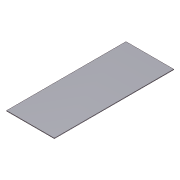
# Autodesk Inventor part: SpaceQuest_interconnect_3
Saved by Autodesk Inventor 2014 SP1 (Build 180222100, 222)
## iProperties
Created: 2013-06-08
Part Number: SpaceQuest_interconnect_3
Material: Stainless Steel
Document SubType Name: Modeling
Designer: Robert Davis
Mass: 0.01616 g
Surface Area: 0.814 cm^2
Volume: 0.002 cm^3
Density: 8.08 g/cm^3
Appearance: Steel
Author: Robert Davis
Autodesk Inventor part; units mm, degrees
ref_plane "YZ Plane" through (0, 0, 0) normal (1, 0, 0) x (0, 1, 0)
ref_plane "XZ Plane" through (0, 0, 0) normal (0, 1, 0) x (-1, 0, 0)
ref_plane "XY Plane" through (0, 0, 0) normal (0, 0, 1) x (1, 0, 0)
sketch "Sketch1" plane through (0, 0, 0) normal (0, 0, 1) x (1, 0, 0)
  line L0 (-2, 5) -> (2, 5)
  line L1 (2, 5) -> (2, -5)
  line L2 (2, -5) -> (-2, -5)
  line L3 (-2, -5) -> (-2, 5)
  line L4 (0, 0) -> (0, 1.6478)
  line L5 (0, 0) -> (2.3787, 0)
  dimension "d0" = 4
  dimension "d1" = 10
  constraints: 12 end point, 3 horizontal, 2 vertical, 1 coincident, 2 other
  measures "d0" distance of L0.start L0.end
  measures "d1" distance of L0.end L1.end
extrude "Extrusion1" add sketch "Sketch1" along normal blind 0.05
body "Solid1"
